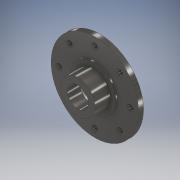
# Autodesk Inventor part: reverse gear lower cylinder cover
Saved by Autodesk Inventor 2017 (Build 210142000, 142)
## iProperties
Created: 2018-11-09
Part Number: reverse gear lower cylinder cover
Material: Generic
Document SubType Name: Modeling
Designer: User
Density: 1 g/cm^3
Appearance: Default
Author: User
Autodesk Inventor part; units mm, degrees
ref_plane "YZ Plane" through (0, 0, 0) normal (1, 0, 0) x (0, 1, 0)
ref_plane "XZ Plane" through (0, 0, 0) normal (0, 1, 0) x (-1, 0, 0)
ref_plane "XY Plane" through (0, 0, 0) normal (0, 0, 1) x (1, 0, 0)
sketch "Sketch1" plane through (0, 0, 0) normal (0, 1, 0) x (-1, 0, 0)
  circle A0 centre (0, 0) radius 27
  dimension "d0" = 54
  constraints: 1 centre point, 1 coincident
  measures "d0" diameter of A0
extrude "Extrusion1" add sketch "Sketch1" along normal blind 3
sketch "Sketch2" plane through (0, 3, 0) normal (0, 1, 0) x (1, 0, 0)
  circle A0 centre (0, 0) radius 16
  dimension "d3" = 32
  constraints: 1 centre point, 1 coincident
  measures "d3" diameter of A0
extrude "Extrusion2" add sketch "Sketch2" along normal blind 1.5
sketch "Sketch3" plane through (0, 0, 0) normal (0, -1, 0) x (1, 0, 0)
  circle A0 centre (0, 0) radius 14
  dimension "d6" = 28
  constraints: 1 centre point, 1 coincident
  measures "d6" diameter of A0
extrude "Extrusion3" add sketch "Sketch3" along normal blind 1
sketch "Sketch4" plane through (0, 4.5, 0) normal (0, 1, 0) x (1, 0, 0)
  circle A0 centre (0, 0) radius 3
  dimension "d9" = 6
  constraints: 1 centre point, 1 coincident
  measures "d9" diameter of A0
extrude "Extrusion4" cut sketch "Sketch4" against normal through all
sketch "Sketch5" plane through (0, -1, 0) normal (0, -1, 0) x (1, 0, 0)
  circle A0 centre (0, 0) radius 6.5
  circle A1 centre (0, 0) radius 10.5
  dimension "d12" = 13
  dimension "d16" = 21
  constraints: 2 centre point, 2 coincident
  measures "d12" diameter of A0
  measures "d16" diameter of A1
extrude "Extrusion6" add sketch "Sketch5" along normal blind 9.5
fillet "Fillet1" radius 2 1 edges at (-6.5, -1, 0)
sketch "Sketch7" plane through (0, 3, 0) normal (0, 1, 0) x (1, 0, 0)
  circle A0 centre (0, 0) radius 3 construction
  circle A1 centre (0, 0) radius 22 construction
  circle A2 centre (-22, 0) radius 1.75
  circle A3 centre (-15.5563, -15.5563) radius 1.75
  circle A4 centre (0, -22) radius 1.75
  circle A5 centre (15.5563, -15.5563) radius 1.75
  circle A6 centre (22, 0) radius 1.75
  circle A7 centre (15.5563, 15.5563) radius 1.75
  circle A8 centre (0, 22) radius 1.75
  circle A9 centre (-15.5563, 15.5563) radius 1.75
  dimension "d20" = 44
  dimension "d22" = 3.5
  dimension "d25" = 360
  constraints: 8 centre point, 1 coincident, 1 horizontal alignment, 19 other
  measures "d22" diameter of A2
extrude "Extrusion7" cut sketch "Sketch7" against normal through all
body "Solid1"
